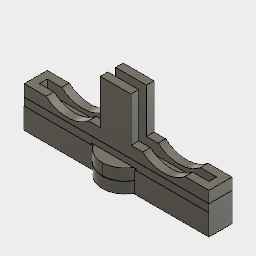
Ultrasonic Stand (Autodesk Fusion 360 design; units mm, degrees)
Autodesk Fusion 360 part; units mm, degrees
sketch "Sketch1" plane through (0, 0, 0) normal (0, 1, 0) x (1, 0, 0)
  circle A0 centre (0, 28) radius 3.95
  circle A1 centre (0, 28) radius 5.95
  dimension "d1" = 7.9
  dimension "d2" = 2
  measures "d1" diameter of A0
extrude "Extrude1" add sketch "Sketch1" along normal blind 3.1 makes body 1
sketch "Sketch2" plane through (0, 0, 0) normal (0, 1, 0) x (1, 0, 0)
  line L0 (-6, 21) -> (6, 21)
  line L1 (6, 21) -> (6, 9)
  line L2 (6, 9) -> (-6, 9)
  line L3 (-6, 9) -> (-6, 21)
  dimension "d5" = 12
  measures "d5" distance of L0.start L0.end
extrude "Extrude2" add sketch "Sketch2" along normal blind 3 separate body makes body 2
fillet "Fillet1" radius 6 4 edges at (-6, 1.5, -21) (-6, 1.5, -9) (6, 1.5, -9) (6, 1.5, -21) on bodies 2
move_body "Move1" bodies 2 to x (1, 0, 0) y (0, 1, 0) z (0, 0, 1) at (0, 2.9, -13)
combine "Combine1" operation add target body 1 tool bodies 2
sketch "Sketch3" plane through (0, 0, 0) normal (0, 1, 0) x (1, 0, 0)
  line L0 (-15, 20) -> (28.9, 20)
  line L1 (28.9, 20) -> (28.9, 18)
  line L2 (28.9, 18) -> (-15, 18)
  line L3 (-15, 18) -> (-15, 20)
  line L4 (29.4, 17.5) -> (-15.5, 17.5)
  line L5 (-15.5, 17.5) -> (-15.5, 20.5)
  line L6 (-15.5, 20.5) -> (29.4, 20.5)
  line L7 (29.4, 20.5) -> (29.4, 17.5)
  dimension "d9" = 43.9
  dimension "d10" = 2
  dimension "d11" = 0.5
  measures "d9" distance of L0.start L0.end
  measures "d10" distance of L0.start L2.end
extrude "Extrude3" add sketch "Sketch3" along normal blind 3 separate body makes body 3
sketch "Sketch4" plane through (0, 0, 0) normal (0, 1, 0) x (1, 0, 0)
  line L0 (-15.5, 20.5) -> (29.3978, 20.5)
  line L1 (29.3978, 20.5) -> (29.3978, 17.5883)
  line L2 (29.3978, 17.5883) -> (-15.5, 17.5883)
  line L3 (-15.5, 17.5883) -> (-15.5, 20.5)
  point P0 (-15.5, 20.5)
  dimension "d14" = 44.8978
  measures "d14" distance of P0 L0.end
extrude "Extrude4" add sketch "Sketch4" against normal blind 2 bodies 3
move_body "Move2" bodies 3 to x (1, 0, 0) y (0, 1, 0) z (0, 0, 1) at (0, 7.5, 0)
move_body "Move3" bodies 3 to x (1, 0, 0) y (0, 1, 0) z (0, 0, 1) at (0, 0, -9)
move_body "Move4" bodies 3 to x (1, 0, 0) y (0, 1, 0) z (0, 0, 1) at (-6, 0, 0)
move_body "Move5" bodies 3 to x (1, 0, 0) y (0, 1, 0) z (0, 0, 1) at (-0.2, 0, 0)
sketch "Sketch5" plane through (0, 0, 0) normal (0, 0, 1) x (1, 0, 0)
  circle A0 centre (13, 17) radius 8.5
  dimension "d17" = 17
  measures "d17" diameter of A0
extrude "Extrude5" cut sketch "Sketch5" against normal blind 40 bodies 3
sketch "Sketch6" plane through (0, 0, 0) normal (0, 0, 1) x (1, 0, 0)
  circle A0 centre (-12, 17) radius 8.5
  dimension "d20" = 17
  measures "d20" diameter of A0
extrude "Extrude6" cut sketch "Sketch6" against normal blind 40 bodies 3
sketch "Sketch7" plane through (0, 0, 0) normal (0, 0, 1) x (1, 0, 0)
  line L0 (2, 23) -> (-2, 23)
  line L1 (-2, 23) -> (-2, 11)
  line L2 (-2, 11) -> (2, 11)
  line L3 (2, 11) -> (2, 23)
  dimension "d23" = 12
  measures "d23" distance of L0.start L2.end
extrude "Extrude7" add sketch "Sketch7" along normal blind 2 separate body makes body 4
shell "Shell1" thickness 2 outward yes removed faces 0 bodies 4
sketch "Sketch8" plane through (0, 0, 0) normal (1, 0, 0) x (0, 0, -1)
  line L0 (0, 30, 6) -> (-2, 30, 6)
  line L1 (-2, 30, 6) -> (-2, 6, 6)
  line L2 (-2, 6, 6) -> (0, 6, 6)
  line L3 (0, 6, 6) -> (0, 30, 6)
extrude "Extrude8" cut sketch "Sketch8" against normal blind 16 contours L0 L1 L2 L3 in plane through (6, 0, 0) normal (1, 0, 0) bodies 4 makes body 5 at (1.3333, 14.3333, 0)
extrude "Extrude9" add 1 faces at (4.8326, 6.5, -29.5) along direction (0, 0, -1) blind 1.5 on bodies 3 bodies 3 1
extrude "Extrude10" add 1 faces at (21.6257, 9.5, -26.5) along direction (0, 0, 1) blind 1.5 on bodies 3 bodies 3
extrude "Extrude11" add 1 faces at (17.4091, 6.3, -26.5883) along direction (0, 0, 1) blind 1.5 on bodies 3 bodies 3
extrude "Extrude12" add 1 faces at (23.2, 9.5, -27) along direction (1, 0, 0) blind 1.5 on bodies 3 bodies 3
extrude "Extrude13" add 1 faces at (23.1978, 6.8333, -29.0294) along direction (1, 0, 0) blind 1.5 on bodies 3 bodies 3
extrude "Extrude14" add 1 faces at (-21.7, 7.8333, -29.0294) along direction (-1, 0, 0) blind 1.5 on bodies 3 bodies 3
extrude "Extrude15" add 1 faces at (18.4091, 6.3, -25.0883) along direction (0, 0, 1) blind 0.1 on bodies 3 bodies 3
move_body "Move6" bodies 4 5 to x (1, 0, 0) y (0, 1, 0) z (0, 0, 1) at (0, 1, -29)
sketch "Sketch9" plane through (0, 0, 0) normal (0, 0, 1) x (1, 0, 0)
  line L0 (24.6978, 5.5) -> (6, 5.5)
  line L1 (6, 5.5) -> (6, 0)
  line L2 (6, 0) -> (24.6978, 0)
  line L3 (24.6978, 0) -> (24.6978, 5.5)
  point P0 (24.6978, 5.5)
  dimension "d44" = 18.6978
  measures "d44" distance of P0 L0.end
extrude "Extrude16" add sketch "Sketch9" along normal blind 6.012 separate body makes body 6
move_body "Move7" bodies 6 to x (1, 0, 0) y (0, 1, 0) z (0, 0, 1) at (0, 0, -31)
copy_body "CopyPasteBodies1" bodies 6 makes body 7
move_body "Move8" bodies 7 to x (1, 0, 0) y (0, 1, 0) z (0, 0, 1) at (-30, 0, 0)
move_body "Move9" bodies 7 to x (1, 0, 0) y (0, 1, 0) z (0, 0, 1) at (0.74, 0, 0)
move_body "Move10" bodies 3 to x (1, 0, 0) y (0, 1, 0) z (0, 0, 1) at (0.5, 0, 0)
extrude "Extrude17" add 1 faces at (24.6978, 1.8333, -28.996) along direction (1, 0, 0) blind 0.5 on bodies 6 bodies 6 4 5 7 3
extrude "Extrude18" cut 1 faces at (-23.26, 3.6667, -28.996) along direction (1, 0, 0) blind 0.5 on bodies 7 bodies 7
move_body "Move11" bodies 4 to x (1, 0, 0) y (0, 1, 0) z (0, 0, 1) at (1, 0, 0)
move_body "Move12" bodies 5 to x (1, 0, 0) y (0, 1, 0) z (0, 0, 1) at (1, 0, 0)
sketch "Sketch10" plane through (0, 0, 0) normal (0, 0, 1) x (1, 0, 0)
  line L0 (-3, 26) -> (8, 26)
  line L1 (8, 26) -> (8, 22)
  line L2 (8, 22) -> (-3, 22)
  line L3 (-3, 22) -> (-3, 26)
  point P0 (-3, 26)
  dimension "d51" = 4
  measures "d51" distance of P0 L2.end
extrude "Extrude19" cut sketch "Sketch10" against normal blind 40 bodies 4 5
combine "Combine2" operation add target body 4 tool bodies 5 6 7
